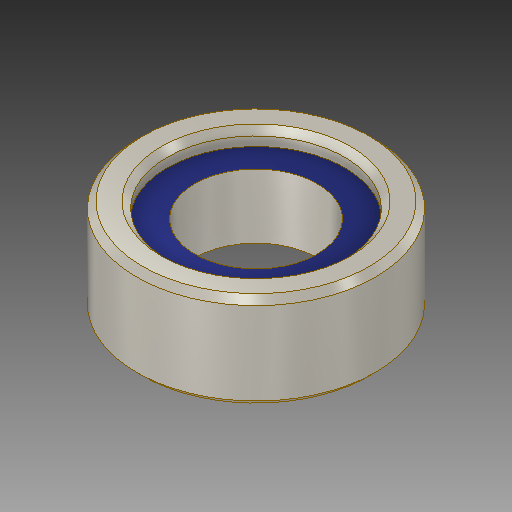
# Autodesk Inventor part: Подшипник 626Z
Saved by Autodesk Inventor 2019 (Build 230136000, 136)
## iProperties
Created: 2019-07-15
Part Number: Подшипник 626Z
Material: Титан
Document SubType Name: Modeling
Designer: user
Density: 4.51 g/cm^3
Appearance: Титан
Description: Подшипник 626Z
Mass: 0.422181 g
Surface Area: 1.80998 cm^2
Volume: 0.09361 cm^3
Author: user
Autodesk Inventor part; units mm, degrees
ref_plane "YZ Plane" through (0, 0, 0) normal (1, 0, 0) x (0, 1, 0)
ref_plane "XZ Plane" through (0, 0, 0) normal (0, 1, 0) x (-1, 0, 0)
ref_plane "XY Plane" through (0, 0, 0) normal (0, 0, 1) x (1, 0, 0)
sketch "Эскиз1" plane through (0, 0, 0) normal (0, 1, 0) x (-1, 0, 0)
  circle A0 centre (0, 0) radius 3.9
  circle A1 centre (0, 0) radius 2
  dimension "d0" = 7.8
  dimension "d1" = 4
  constraints: 2 centre point, 1 coincident
  measures "d0" diameter of A0
  measures "d1" diameter of A1
extrude "Выдавливание1" add sketch "Эскиз1" along normal blind 3.1
sketch "Эскиз2" plane through (0, 3.1, 0) normal (0, 1, 0) x (1, 0, 0)
  circle A0 centre (0, 0) radius 3
  circle A1 centre (0, 0) radius 2.9
  circle A2 centre (0, 0) radius 3.9 projected
  circle A3 centre (0, 0) radius 2 projected
  dimension "d4" = 1
  dimension "d5" = 1
  constraints: 2 centre point, 2 coincident
  measures "d4" radial gap between concentric circles of A1 A2
  measures "d5" radial gap between concentric circles of A3 A0
extrude "Выдавливание2" cut sketch "Эскиз2" against normal blind 0.5 contours A1 | A3
sketch "Эскиз3" plane through (0, 0, 0) normal (0, -1, 0) x (1, 0, 0)
  circle A0 centre (0, 0) radius 2.9 projected
  circle A1 centre (0, 0) radius 3
  circle A2 centre (0, 0) radius 2.9
  circle A3 centre (0, 0) radius 3.9
  circle A4 centre (0, 0) radius 2
  dimension "d13" = 1
  dimension "d14" = 1
  constraints: 4 centre point, 2 coincident
  measures "d13" radial gap between concentric circles of A2 A3
  measures "d14" radial gap between concentric circles of A4 A1
extrude "Выдавливание3" cut sketch "Эскиз3" against normal blind 0.5 contours A0 | A4
chamfer "Фаска1" distance 0.2 angle 45 4 edges at (-2.9, 0, 0) (3.9, 0, 0) (3.9, 3.1, 0) (-2.9, 3.1, 0)
